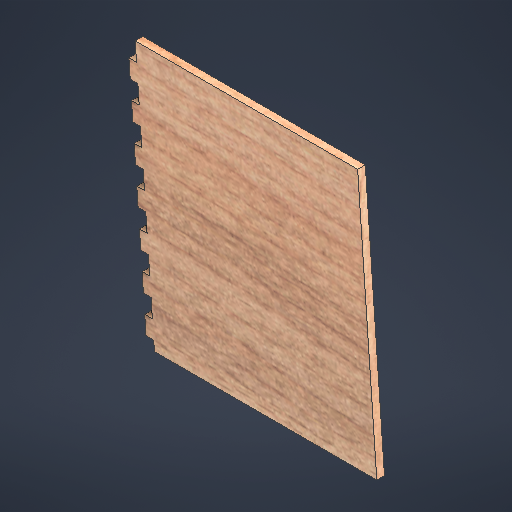
# Autodesk Inventor part: стульчак 3
Saved by Autodesk Inventor 2025 (Build 290162000, 162)
## iProperties
Created: 2025-01-28
Part Number: стульчак 3
Material: Древесина (береза)
Document SubType Name: Modeling
Designer: GameHD
Density: 0.55 g/cm^3
Appearance: Береза — натуральный — полированный
Author: GameHD
Autodesk Inventor part; units mm, degrees
ref_plane "YZ Plane" through (0, 0, 0) normal (1, 0, 0) x (0, 1, 0)
ref_plane "XZ Plane" through (0, 0, 0) normal (0, 1, 0) x (-1, 0, 0)
ref_plane "XY Plane" through (0, 0, 0) normal (0, 0, 1) x (1, 0, 0)
sketch "Эскиз1" plane through (0, 0, 0) normal (0, 0, 1) x (1, 0, 0)
  line L0 (-60, -75) -> (60, -75)
  line L1 (60, -75) -> (60, 75)
  line L2 (60, 75) -> (-60, 75)
  line L3 (-60, 75) -> (-60, -75)
  line L4 (-60, -75) -> (60, 75) construction
  line L5 (60, -75) -> (-60, 75) construction
  point P0 (0, 0)
  dimension "d2" = 150
  dimension "d3" = 120
  constraints: 12 end point, 2 midpoint, 2 parallel, 1 horizontal, 1 perpendicular
  measures "d2" distance of L2.end L0.start
  measures "d3" distance of L1.end L2.end
extrude "Выдавливание1" add sketch "Эскиз1" along normal blind 4
sketch "Эскиз2" plane through (0, 0, 4) normal (0, 0, 1) x (1, 0, 0)
  line L0 (-56, -45) -> (-60, -45)
  line L1 (-60, -55) -> (-60, -45)
  line L2 (-60, -55) -> (-56, -55)
  line L3 (-56, -45) -> (-56, -55)
  line L4 (-56, -55) -> (-56, -65)
  line L5 (-60, -55) -> (-56, -55)
  line L6 (-60, -65) -> (-60, -55)
  line L7 (-60, -65) -> (-56, -65)
  line L8 (-56, -65) -> (-60, -65)
  line L9 (-60, -70.3625) -> (-60, -65)
  line L10 (-60, -70.3625) -> (-56, -70.3625)
  line L11 (-56, -65) -> (-56, -70.3625)
  line L12 (-56, -35) -> (-56, -45)
  line L13 (-60, -35) -> (-56, -35)
  line L14 (-60, -45) -> (-60, -35)
  line L15 (-60, -45) -> (-56, -45)
  line L16 (-56, -25) -> (-60, -25)
  line L17 (-60, -35) -> (-60, -25)
  line L18 (-60, -35) -> (-56, -35)
  line L19 (-56, -25) -> (-56, -35)
  line L20 (-56, -15) -> (-56, -25)
  line L21 (-60, -15) -> (-56, -15)
  line L22 (-60, -25) -> (-60, -15)
  line L23 (-60, -25) -> (-56, -25)
  line L24 (-56, -12) -> (-60, -12)
  line L25 (-60, -15) -> (-56, -15)
  line L26 (-56, -5) -> (-56, -15)
  line L27 (-56, -5) -> (-60, -5)
  line L28 (-60, -15) -> (-60, -5)
  line L29 (-56, 5) -> (-56, -5)
  line L30 (-60, 5) -> (-56, 5)
  line L31 (-60, -5) -> (-60, 5)
  line L32 (-60, -5) -> (-56, -5)
  line L33 (-60, 5) -> (-56, 5)
  line L34 (-56, 15) -> (-56, 5)
  line L35 (-56, 15) -> (-60, 15)
  line L36 (-60, 5) -> (-60, 15)
  line L37 (-56, 25) -> (-56, 15)
  line L38 (-60, 25) -> (-56, 25)
  line L39 (-60, 15) -> (-60, 25)
  line L40 (-60, 15) -> (-56, 15)
  line L41 (-56, 35) -> (-60, 35)
  line L42 (-60, 25) -> (-60, 35)
  line L43 (-60, 25) -> (-56, 25)
  line L44 (-56, 35) -> (-56, 25)
  line L45 (-56, 45) -> (-56, 35)
  line L46 (-60, 45) -> (-56, 45)
  line L47 (-60, 35) -> (-60, 45)
  line L48 (-60, 35) -> (-56, 35)
  line L49 (-56, 55) -> (-60, 55)
  line L50 (-60, 45) -> (-60, 55)
  line L51 (-60, 45) -> (-56, 45)
  line L52 (-56, 55) -> (-56, 45)
  line L53 (-56, 65) -> (-56, 55)
  line L54 (-60, 65) -> (-56, 65)
  line L55 (-60, 55) -> (-60, 65)
  line L56 (-60, 55) -> (-56, 55)
  line L57 (-60, 65) -> (-56, 65)
  line L58 (-56, 75) -> (-56, 65)
  line L59 (-56, 75) -> (-60, 75)
  line L60 (-60, 65) -> (-60, 75)
  line L61 (60, -75) -> (60, 75) projected
  line L62 (60, 75) -> (-60, 75) projected
  line L63 (-60, 75) -> (-60, -75) projected
  line L64 (-60, -75) -> (60, -75) projected
  line L65 (-60, -70.3625) -> (123.825, -70.3625)
  line L66 (123.825, -70.3625) -> (123.825, -115.8875)
  line L67 (123.825, -115.8875) -> (-60, -115.8875)
  line L68 (-60, -115.8875) -> (-60, -70.3625)
  point P0 (0, 0)
  point P1 (-56, -27.5)
  constraints: 130 end point, 2 parallel, 1 horizontal, 1 perpendicular
extrude "Выдавливание2" cut sketch "Эскиз2" against normal blind 10 contours L3 L2 L1 L0 | L13 L17 L16 L19 | L11 L10 L9 L7 | L65 L61 L64 L63 L10 | L21 L28 L24 L26 | L65 L66 L67 L68 L64 L61 | L24 L28 L27 L26 | L58 L54 L60 L59 | L30 L36 L35 L34 | L52 L46 L50 L49 | L38 L42 L41 L44
sketch "Эскиз3" plane through (60, 75, 4) normal (1, 0, 0) x (0, 0, -1)
  line L0 (0, 0) -> (0, -10) projected
  line L1 (4, 0) -> (0, 0) projected
  line L2 (0, -145.3625) -> (4, -145.3625) projected
  line L3 (4, -145.3625) -> (4, 0) projected
  line L4 (4, 0) -> (0, 0) projected
  line L5 (0, -145.3625) -> (0, 0) projected
  line L6 (14, 0) -> (14, -145.3625)
  line L7 (14, -145.3625) -> (0, -145.3625)
  line L8 (0, -145.3625) -> (0, 0)
  line L9 (14, 0) -> (10, 0)
  line L10 (10, 0) -> (0, -145.3625)
  line L11 (-4, 0) -> (0, 0)
  line L12 (0, -145.3625) -> (-4, -145.3625)
  line L13 (-4, -145.3625) -> (-4, 0)
  line L14 (-4, 0) -> (0, 0)
  line L15 (-14, 0) -> (-14, -145.3625)
  line L16 (-14, -145.3625) -> (0, -145.3625)
  line L17 (-14, 0) -> (-10, 0)
  line L18 (-10, 0) -> (0, -145.3625)
  point P0 (4, -75)
  point P1 (-4, -75)
  point P2 (-4, -87.2175)
  dimension "d6" = 14
  dimension "d7" = 14
  dimension "d14" = 4
  constraints: 26 end point, 7 symmetric about line, 1 horizontal, 1 perpendicular, 1 vertical
  measures "d6" distance of L0.start L6.start
  measures "d7" distance of L6.end L7.end
  measures "d14" distance of L6.start L9.end
extrude "Выдавливание3" add sketch "Эскиз3" against normal up to surface (120 mm away) contours L12 L13 L18 | L13 L16 L15 L17 L18
sketch "Эскиз4" plane through (0, 0, 4) normal (0, 0, 1) x (1, 0, 0)
  line L0 (-56, -35) -> (-60, -35) projected
  line L1 (-60, -35) -> (-60, -45) projected
  line L2 (-60, -45) -> (-56, -45) projected
  line L3 (-56, -45) -> (-56, -55) projected
  line L4 (-56, -55) -> (-60, -55) projected
  line L5 (-60, -55) -> (-60, -65) projected
  line L6 (-60, -65) -> (-56, -65) projected
  line L7 (-56, -65) -> (-56, -70.3625) projected
  line L8 (-56, -70.3625) -> (60, -70.3625) projected
  line L9 (60, -70.3625) -> (60, 75) projected
  line L10 (60, 75) -> (-56, 75) projected
  line L11 (-56, 75) -> (-56, 65) projected
  line L12 (-56, 65) -> (-60, 65) projected
  line L13 (-60, 65) -> (-60, 55) projected
  line L14 (-60, 55) -> (-56, 55) projected
  line L15 (-56, 55) -> (-56, 45) projected
  line L16 (-56, 45) -> (-60, 45) projected
  line L17 (-60, 45) -> (-60, 35) projected
  line L18 (-60, 35) -> (-56, 35) projected
  line L19 (-56, 35) -> (-56, 25) projected
  line L20 (-56, 25) -> (-60, 25) projected
  line L21 (-60, 25) -> (-60, 15) projected
  line L22 (-60, 15) -> (-56, 15) projected
  line L23 (-56, 15) -> (-56, 5) projected
  line L24 (-56, 5) -> (-60, 5) projected
  line L25 (-60, 5) -> (-60, -5) projected
  line L26 (-60, -5) -> (-56, -5) projected
  line L27 (-56, -5) -> (-56, -15) projected
  line L28 (-56, -15) -> (-60, -15) projected
  line L29 (-60, -15) -> (-60, -25) projected
  line L30 (-60, -25) -> (-56, -25) projected
  line L31 (-56, -25) -> (-56, -35) projected
  line L32 (60, 75) -> (-87.3125, 75)
  line L33 (-87.3125, 75) -> (-87.3125, -70.3625)
  line L34 (-87.3125, -70.3625) -> (60, -70.3625)
  line L35 (60, -70.3625) -> (60, 75)
  point P0 (0, 0)
  constraints: 8 end point, 2 parallel, 1 horizontal, 1 perpendicular
extrude "Выдавливание4" cut sketch "Эскиз4" along normal through all contours L0 L1 L2 L3 L4 L5 L6 L7 L34 L33 L32 L11 L12 L13 L14 L15 L16 L17 L18 L19 L20 L21 L22 L23 L24 L25 L26 L27 L28 L29 L30 L31
sketch "Эскиз5" plane through (60, -70.3625, 4) normal (1, 0, 0) x (0, 0, -1)
  line L0 (0, 0) -> (0, 145.3625) projected
  line L1 (0, 0) -> (4, 0) projected
  line L2 (4, 0) -> (4, 145.3625) projected
  line L3 (4, 145.3625) -> (0, 145.3625) projected
extrude "Выдавливание5" cut sketch "Эскиз5" against normal through all
sketch "Эскиз6" plane through (-60, -25, 18) normal (-1, 0, 0) x (0, 0, 1)
  line L0 (-4, 100) -> (0, 100) projected
  line L1 (0, -45.3625) -> (-14, -45.3625) projected
  line L2 (-4, 100) -> (-14, -45.3625)
  line L3 (-14, -45.3625) -> (-10, -45.3625)
  line L4 (-10, -45.3625) -> (0, 100)
  line L5 (0, 100) -> (0, -45.3625)
  line L6 (-13.6311, -40) -> (0, -40) projected
  line L7 (-10, -45.3625) -> (0, -45.3625)
  point P0 (-18, 25)
  dimension "d15" = 4
  constraints: 10 end point, 1 collinear, 1 parallel, 1 perpendicular, 1 point on line
  measures "d15" distance of L1.end L3.end
extrude "Выдавливание6" cut sketch "Эскиз6" against normal through all contours L5 L6 L4 | L6 L5 L1 L4
